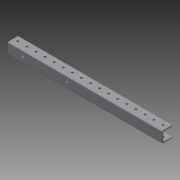
# Autodesk Inventor part: c-channel
Saved by Autodesk Inventor 2015 SP1 (Build 190203100, 203)
## iProperties
Created: 2015-01-13
Part Number: c-channel
Material: Generic
Document SubType Name: Modeling
Designer: Jarod
Density: 1 g/cm^3
Appearance: Default
Author: Jarod
Autodesk Inventor part; units mm, degrees
ref_plane "YZ Plane" through (0, 0, 0) normal (1, 0, 0) x (0, 1, 0)
ref_plane "XZ Plane" through (0, 0, 0) normal (0, 1, 0) x (-1, 0, 0)
ref_plane "XY Plane" through (0, 0, 0) normal (0, 0, 1) x (1, 0, 0)
sketch "Sketch1" plane through (0, 0, 0) normal (1, 0, 0) x (0, 1, 0)
  line L0 (0, 0) -> (0, 25.4)
  line L1 (3.175, 28.575) -> (28.575, 28.575)
  line L2 (31.75, 25.4) -> (31.75, 0)
  line L3 (28.575, 0) -> (28.575, 25.4)
  line L4 (28.575, 25.4) -> (3.175, 25.4)
  line L5 (3.175, 25.4) -> (3.175, 0)
  line L6 (0, 0) -> (3.175, 0)
  line L7 (28.575, 0) -> (31.75, 0)
  arc A0 (3.175, 28.575) -> (0, 25.4) centre (3.175, 25.4) ccw
  arc A1 (31.75, 25.4) -> (28.575, 28.575) centre (28.575, 25.4) ccw
  point P0 (0, 28.575)
  point P1 (31.75, 28.575)
  dimension "d0" = 28.575
  dimension "d2" = 31.75
  dimension "d3" = 90
  dimension "d4" = 28.575
  dimension "d5" = 90
  dimension "d6" = 3.175
  dimension "d7" = 3.175
  constraints: 16 end point, 4 perpendicular, 4 point on circle, 4 point on line, 4 tangent, 2 centre point, 1 collinear, 1 equal radius, 1 horizontal, 1 vertical, 2 other
  measures "d0" distance of L0.start point (0, 28.575)
  measures "d2" distance of point (0, 28.575) point (31.75, 28.575)
  measures "d3" angle of L0 L1
  measures "d4" distance of point (31.75, 28.575) L2.end
  measures "d5" angle of L1 L2
  measures "d6" distance between parallel lines of L1 L4
  measures "d7" radius of A0
extrude "Extrusion1" add sketch "Sketch1" along normal blind 406.4
sketch "Sketch2" plane through (0, 31.75, 25.4) normal (0, 1, 0) x (1, 0, 0)
  line L0 (0, 0) -> (0, 25.4) projected
  line L1 (0, 0) -> (406.4, 0) projected
  line L2 (406.4, 25.4) -> (406.4, 0) projected
  line L3 (0, 25.4) -> (406.4, 25.4) projected
  point P0 (0, 25.4)
  point P1 (12.7, 12.7)
  dimension "d10" = 12.7
  dimension "d11" = 12.7
  measures "d10" distance from line of L0 point (12.7, 12.7)
  measures "d11" distance from line of L3 point (12.7, 12.7)
hole "Hole1" at (12.7, 31.75, 12.7) direction (0, -1, 0) diameter 6.35 end through all
pattern_linear "Rectangular Pattern1" count 20 spacing 25.4 along (1, 0, 0) of "Hole1"
sketch "Sketch4" plane through (0, 3.175, 28.575) normal (0, 0, 1) x (1, 0, 0)
  line L0 (0, 0) -> (0, 25.4) projected
  line L1 (0, -3.175) -> (0, 0) projected
  line L2 (0, -3.175) -> (406.4, -3.175) projected
  line L3 (406.4, 0) -> (406.4, -3.175) projected
  line L4 (0, 0) -> (406.4, 0) projected
  point P0 (0, -3.175)
  point P1 (15.875, 14.2875)
  point P2 (139.7, 14.2875)
  dimension "d28" = 15.875
  dimension "d30" = 139.7
  dimension "d45" = 17.4625
  dimension "d46" = 17.4625
  measures "d28" distance from line of L0 point (15.875, 14.287)
  measures "d30" distance from line of L0 point (139.7, 14.287)
  measures "d45" distance from line of L2 point (15.875, 14.287)
  measures "d46" distance from line of L2 point (139.7, 14.287)
hole "Hole2" at (15.875, 17.4625, 28.575) at (139.7, 17.4625, 28.575) direction (0, 0, -1) diameter 6.35 end through all
sketch "Sketch5" plane through (0, 0, 0) normal (-1, 0, 0) x (0, 0, 1)
  line L0 (0, 0) -> (25.4, 0) projected
  arc A0 (25.4, 0) -> (28.575, 3.175) centre (25.4, 3.175) ccw projected
  line L1 (28.575, 3.175) -> (28.575, 28.575) projected
  arc A1 (28.575, 28.575) -> (25.4, 31.75) centre (25.4, 28.575) ccw projected
  line L2 (25.4, 31.75) -> (0, 31.75) projected
  line L3 (0, 31.75) -> (0, 28.575) projected
  line L4 (0, 28.575) -> (25.4, 28.575) projected
  line L5 (25.4, 28.575) -> (25.4, 3.175) projected
  line L6 (25.4, 3.175) -> (0, 3.175)
  line L7 (0, 3.175) -> (0, 0)
  line L8 (0, 0) -> (25.4, 0)
  line L9 (25.4, 0) -> (25.4, 3.175)
  constraints: 8 end point, 2 parallel, 1 horizontal, 1 perpendicular
extrude "Extrusion3" add sketch "Sketch5" along normal blind 25.4 contours L9 L5 L4 L3 L2 A1 L1 A0
sketch "Sketch6" plane through (406.4, 31.75, 25.4) normal (0, 1, 0) x (1, 0, 0)
  line L0 (0, 25.4) -> (-431.8, 25.4) projected
  line L1 (-431.8, 0) -> (-431.8, 25.4) projected
  circle A0 centre (-419.1, 12.7) radius 3.175
  point P0 (-406.4, 25.4)
  dimension "d40" = 6.35
  dimension "d41" = 12.7
  dimension "d42" = 12.7
  constraints: 1 centre point
  measures "d40" diameter of A0
  measures "d41" distance from line of L0 A0.centre
  measures "d42" distance from line of L1 A0.centre
extrude "Extrusion4" cut sketch "Sketch6" against normal blind 25.4
fillet "Fillet1" radius 3.175 2 edges at (203.2, 3.175, 25.4) (190.5, 28.575, 25.4)
body "Solid1"
